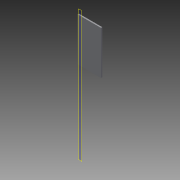
# Autodesk Inventor part: Aluminum Final Mounting Plate
Saved by Autodesk Inventor 2015 (Build 190159000, 159)
## iProperties
Created: 2015-01-28
Part Number: Aluminum Final Mounting Plate
Material: Generic
Document SubType Name: Modeling
Designer: jhirshland1
Density: 1 g/cm^3
Appearance: Default
Author: jhirshland1
Autodesk Inventor part; units mm, degrees
ref_plane "YZ Plane" through (0, 0, 0) normal (1, 0, 0) x (0, 1, 0)
ref_plane "XZ Plane" through (0, 0, 0) normal (0, 1, 0) x (-1, 0, 0)
ref_plane "XY Plane" through (0, 0, 0) normal (0, 0, 1) x (1, 0, 0)
ref_plane "Work Plane1" through (45.1427, 7.5316, -333.0131) normal (-0.0001, 0, -1) x (0, -1, 0)
sketch "Sketch1" plane through (45.1427, 7.5316, -333.0131) normal (-0.0001, 0, -1) x (0, -1, 0)
  line L0 (333.4019, -100.965) -> (333.4019, -89.027) projected
  line L1 (117.2921, 3.175) -> (326.375, 3.175)
  line L2 (326.375, 3.175) -> (326.375, -108.4168)
  line L3 (326.375, -108.4168) -> (117.2921, -108.4168)
  line L4 (117.2921, -108.4168) -> (117.2921, 3.175)
  circle A0 centre (673.1, -9.525) radius 2.667 projected
  circle A1 centre (647.7, -9.525) radius 2.667 projected
  circle A2 centre (622.3, -9.525) radius 2.667 projected
  circle A3 centre (596.9, -9.525) radius 2.667 projected
  circle A4 centre (571.5, -9.525) radius 2.667 projected
  circle A5 centre (546.1, -9.525) radius 2.667 projected
  circle A6 centre (520.7, -9.525) radius 2.667 projected
  circle A7 centre (495.3, -9.525) radius 2.667 projected
  circle A8 centre (469.9, -9.525) radius 2.667 projected
  circle A9 centre (444.5, -9.525) radius 2.667 projected
  circle A10 centre (419.1, -9.525) radius 2.667 projected
  circle A11 centre (393.7, -9.525) radius 2.667 projected
  circle A12 centre (368.3, -9.525) radius 2.667 projected
  circle A13 centre (342.9, -9.525) radius 2.667 projected
  circle A14 centre (317.5, -9.525) radius 2.667 projected
  circle A15 centre (292.1, -9.525) radius 2.667 projected
  circle A16 centre (266.7, -9.525) radius 2.667 projected
  circle A17 centre (241.3, -9.525) radius 2.667 projected
  circle A18 centre (215.9, -9.525) radius 2.667 projected
  circle A19 centre (190.5, -9.525) radius 2.667 projected
  circle A20 centre (165.1, -9.525) radius 2.667 projected
  circle A21 centre (139.7, -9.525) radius 2.667 projected
  line L5 (692.3329, -15.875) -> (692.3329, -0.762) projected
  line L6 (120.4671, -0.762) -> (692.3329, -0.762) projected
  line L7 (120.4671, -0.762) -> (120.4671, -15.875) projected
  line L8 (120.4671, -15.875) -> (692.3329, -15.875) projected
  line L9 (121.2291, -672.465) -> (136.3421, -672.465) projected
  line L10 (136.3421, -672.465) -> (136.3421, -19.685) projected
  line L11 (136.3421, -19.685) -> (121.2291, -19.685) projected
  line L12 (121.2291, -672.465) -> (121.2291, -19.685) projected
  circle A22 centre (129.9921, -663.575) radius 2.667 projected
  circle A23 centre (129.9921, -638.175) radius 2.667 projected
  circle A24 centre (129.9921, -612.775) radius 2.667 projected
  circle A25 centre (129.9921, -587.375) radius 2.667 projected
  circle A26 centre (129.9921, -561.975) radius 2.667 projected
  circle A27 centre (129.9921, -536.575) radius 2.667 projected
  circle A28 centre (129.9921, -511.175) radius 2.667 projected
  circle A29 centre (129.9921, -485.775) radius 2.667 projected
  circle A30 centre (129.9921, -460.375) radius 2.667 projected
  circle A31 centre (129.9921, -434.975) radius 2.667 projected
  circle A32 centre (129.9921, -409.575) radius 2.667 projected
  circle A33 centre (129.9921, -384.175) radius 2.667 projected
  circle A34 centre (129.9921, -358.775) radius 2.667 projected
  circle A35 centre (129.9921, -333.375) radius 2.667 projected
  circle A36 centre (129.9921, -307.975) radius 2.667 projected
  circle A37 centre (129.9921, -282.575) radius 2.667 projected
  circle A38 centre (129.9921, -257.175) radius 2.667 projected
  circle A39 centre (129.9921, -231.775) radius 2.667 projected
  circle A40 centre (129.9921, -206.375) radius 2.667 projected
  circle A41 centre (129.9921, -180.975) radius 2.667 projected
  circle A42 centre (129.9921, -155.575) radius 2.667 projected
  circle A43 centre (129.9921, -130.175) radius 2.667 projected
  circle A44 centre (129.9921, -104.775) radius 2.667 projected
  circle A45 centre (129.9921, -79.375) radius 2.667 projected
  circle A46 centre (129.9921, -53.975) radius 2.667 projected
  circle A47 centre (129.9921, -28.575) radius 2.667 projected
  circle A48 centre (180.3669, -28.575) radius 2.667 projected
  circle A49 centre (180.3669, -53.975) radius 2.667 projected
  circle A50 centre (180.3669, -79.375) radius 2.667 projected
  circle A51 centre (180.3669, -104.775) radius 2.667 projected
  circle A52 centre (180.3669, -130.175) radius 2.667 projected
  circle A53 centre (180.3669, -155.575) radius 2.667 projected
  circle A54 centre (180.3669, -180.975) radius 2.667 projected
  circle A55 centre (180.3669, -206.375) radius 2.667 projected
  circle A56 centre (180.3669, -231.775) radius 2.667 projected
  circle A57 centre (180.3669, -257.175) radius 2.667 projected
  circle A58 centre (180.3669, -282.575) radius 2.667 projected
  line L13 (192.3049, -15.875) -> (174.0169, -15.875) projected
  line L14 (174.0169, -15.875) -> (174.0169, -292.1) projected
  line L15 (174.0169, -292.1) -> (177.1919, -295.275) projected
  line L16 (192.3049, -295.275) -> (177.1919, -295.275) projected
  line L17 (192.3049, -15.875) -> (192.3049, -295.275) projected
  circle A59 centre (219.1019, -72.39) radius 2.667 projected
  circle A60 centre (244.5019, -72.39) radius 2.667 projected
  circle A61 centre (269.9019, -72.39) radius 2.667 projected
  circle A62 centre (295.3019, -72.39) radius 2.667 projected
  circle A63 centre (320.7019, -72.39) radius 2.667 projected
  circle A64 centre (346.1019, -72.39) radius 2.667 projected
  line L18 (212.1169, -66.04) -> (212.1169, -84.328) projected
  line L19 (358.8019, -84.328) -> (212.1169, -84.328) projected
  line L20 (358.8019, -84.328) -> (358.8019, -69.215) projected
  line L21 (358.8019, -69.215) -> (355.6269, -66.04) projected
  line L22 (355.6269, -66.04) -> (212.1169, -66.04) projected
  point P0 (7.5323, 45.1616)
  constraints: 8 end point, 2 parallel, 1 horizontal, 1 perpendicular, 1 other
extrude "Extrusion1" add sketch "Sketch1" along normal blind 6.35 contours L1 L2 L6 L7 L8 L14 L3 L10 L11 L12 L4 | L2 L8 L7 L6 | L12 L11 L10 L3 | L2 L22 L18 L19 L3 L17 L8 | L2 L19 L18 L22 | L17 L3 L14 L8 | A14 | A15 | A16 | A17 | A18 | A19 | A20 | A21 | A44 | A45 | A46 | A47 | A48 | A49 | A50 | A51 | A59 | A60 | A61 | A62 | A63
sketch "Sketch2" plane through (45.1423, 7.5316, -339.3631) normal (-0.0001, 0, -1) x (-1, 0, 0.0001)
  circle A0 centre (-9.525, -673.1) radius 2.667 projected
  circle A1 centre (-9.525, -647.7) radius 2.667 projected
  circle A2 centre (-9.525, -622.3) radius 2.667 projected
  circle A3 centre (-9.525, -596.9) radius 2.667 projected
  circle A4 centre (-9.525, -571.5) radius 2.667 projected
  circle A5 centre (-9.525, -546.1) radius 2.667 projected
  circle A6 centre (-9.525, -520.7) radius 2.667 projected
  circle A7 centre (-9.525, -495.3) radius 2.667 projected
  circle A8 centre (-9.525, -469.9) radius 2.667 projected
  circle A9 centre (-9.525, -444.5) radius 2.667 projected
  circle A10 centre (-9.525, -419.1) radius 2.667 projected
  circle A11 centre (-9.525, -393.7) radius 2.667 projected
  circle A12 centre (-9.525, -368.3) radius 2.667 projected
  circle A13 centre (-9.525, -342.9) radius 2.667 projected
  circle A14 centre (-9.525, -317.5) radius 2.667 projected
  circle A15 centre (-9.525, -292.1) radius 2.667 projected
  circle A16 centre (-9.525, -266.7) radius 2.667 projected
  circle A17 centre (-9.525, -241.3) radius 2.667 projected
  circle A18 centre (-9.525, -215.9) radius 2.667 projected
  circle A19 centre (-9.525, -190.5) radius 2.667 projected
  circle A20 centre (-9.525, -165.1) radius 2.667 projected
  circle A21 centre (-9.525, -139.7) radius 2.667 projected
  line L0 (-15.875, -692.3329) -> (-0.762, -692.3329) projected
  line L1 (-0.762, -120.4671) -> (-0.762, -692.3329) projected
  line L2 (-0.762, -120.4671) -> (-15.875, -120.4671) projected
  line L3 (-15.875, -120.4671) -> (-15.875, -692.3329) projected
  circle A22 centre (-72.39, -219.1019) radius 2.667 projected
  circle A23 centre (-72.39, -244.5019) radius 2.667 projected
  circle A24 centre (-72.39, -269.9019) radius 2.667 projected
  circle A25 centre (-72.39, -295.3019) radius 2.667 projected
  circle A26 centre (-72.39, -320.7019) radius 2.667 projected
  circle A27 centre (-72.39, -346.1019) radius 2.667 projected
  line L4 (-66.04, -212.1169) -> (-84.328, -212.1169) projected
  line L5 (-84.328, -358.8019) -> (-84.328, -212.1169) projected
  line L6 (-84.328, -358.8019) -> (-69.215, -358.8019) projected
  line L7 (-69.215, -358.8019) -> (-66.04, -355.6269) projected
  line L8 (-66.04, -355.6269) -> (-66.04, -212.1169) projected
  circle A28 centre (-28.575, -180.3669) radius 2.667 projected
  circle A29 centre (-53.975, -180.3669) radius 2.667 projected
  circle A30 centre (-79.375, -180.3669) radius 2.667 projected
  circle A31 centre (-104.775, -180.3669) radius 2.667 projected
  circle A32 centre (-130.175, -180.3669) radius 2.667 projected
  circle A33 centre (-155.575, -180.3669) radius 2.667 projected
  circle A34 centre (-180.975, -180.3669) radius 2.667 projected
  circle A35 centre (-206.375, -180.3669) radius 2.667 projected
  circle A36 centre (-231.775, -180.3669) radius 2.667 projected
  circle A37 centre (-257.175, -180.3669) radius 2.667 projected
  circle A38 centre (-282.575, -180.3669) radius 2.667 projected
  line L9 (-15.875, -192.3049) -> (-15.875, -174.0169) projected
  line L10 (-15.875, -174.0169) -> (-292.1, -174.0169) projected
  line L11 (-292.1, -174.0169) -> (-295.275, -177.1919) projected
  line L12 (-295.275, -192.3049) -> (-295.275, -177.1919) projected
  line L13 (-15.875, -192.3049) -> (-295.275, -192.3049) projected
  line L14 (-672.465, -121.2291) -> (-672.465, -136.3421) projected
  line L15 (-672.465, -136.3421) -> (-19.685, -136.3421) projected
  line L16 (-19.685, -136.3421) -> (-19.685, -121.2291) projected
  line L17 (-672.465, -121.2291) -> (-19.685, -121.2291) projected
  circle A39 centre (-663.575, -129.9921) radius 2.667 projected
  circle A40 centre (-638.175, -129.9921) radius 2.667 projected
  circle A41 centre (-612.775, -129.9921) radius 2.667 projected
  circle A42 centre (-587.375, -129.9921) radius 2.667 projected
  circle A43 centre (-561.975, -129.9921) radius 2.667 projected
  circle A44 centre (-536.575, -129.9921) radius 2.667 projected
  circle A45 centre (-511.175, -129.9921) radius 2.667 projected
  circle A46 centre (-485.775, -129.9921) radius 2.667 projected
  circle A47 centre (-460.375, -129.9921) radius 2.667 projected
  circle A48 centre (-434.975, -129.9921) radius 2.667 projected
  circle A49 centre (-409.575, -129.9921) radius 2.667 projected
  circle A50 centre (-384.175, -129.9921) radius 2.667 projected
  circle A51 centre (-358.775, -129.9921) radius 2.667 projected
  circle A52 centre (-333.375, -129.9921) radius 2.667 projected
  circle A53 centre (-307.975, -129.9921) radius 2.667 projected
  circle A54 centre (-282.575, -129.9921) radius 2.667 projected
  circle A55 centre (-257.175, -129.9921) radius 2.667 projected
  circle A56 centre (-231.775, -129.9921) radius 2.667 projected
  circle A57 centre (-206.375, -129.9921) radius 2.667 projected
  circle A58 centre (-180.975, -129.9921) radius 2.667 projected
  circle A59 centre (-155.575, -129.9921) radius 2.667 projected
  circle A60 centre (-130.175, -129.9921) radius 2.667 projected
  circle A61 centre (-104.775, -129.9921) radius 2.667 projected
  circle A62 centre (-79.375, -129.9921) radius 2.667 projected
  circle A63 centre (-53.975, -129.9921) radius 2.667 projected
  circle A64 centre (-28.575, -129.9921) radius 2.667 projected
  point P0 (45.1616, -7.5323)
extrude "Extrusion2" cut sketch "Sketch2" along normal mid plane 6.35 contours A14 | A15 | A16 | A17 | A18 | A19 | A20 | A21 | A22 | A23 | A24 | A25 | A26 | A28 | A29 | A30 | A31 | A61 | A62 | A63 | A64
body "Solid1"
